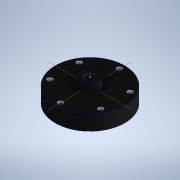
# Autodesk Inventor part: valve housing
Saved by Autodesk Inventor 2021.1 (Build 251245000, 245)
## iProperties
Created: 2020-08-29
Part Number: valve housing
Material: Aluminum 6061
Document SubType Name: Sheet Metal
Designer: Vamshi
Mass: 6082.64 g
Surface Area: 1279.34 cm^2
Volume: 2252.83 cm^3
Density: 2.7 g/cm^3
Sheet Metal Rule: Default
Appearance: Aluminum - Flat
Author: Vamshi
Autodesk Inventor part; units mm, degrees
ref_plane "YZ Plane" through (0, 0, 0) normal (1, 0, 0) x (0, 1, 0)
ref_plane "XZ Plane" through (0, 0, 0) normal (0, 1, 0) x (-1, 0, 0)
ref_plane "XY Plane" through (0, 0, 0) normal (0, 0, 1) x (1, 0, 0)
sketch "Sketch1" plane through (0, 0, 0) normal (0, 0, 1) x (1, 0, 0)
  circle A0 centre (0, 0) radius 116.84
  circle A1 centre (0, 0) radius 30.48
  dimension "d0" = 233.68
  dimension "d1" = 60.96
  constraints: 2 centre point, 2 coincident
  measures "d0" diameter of A0
  measures "d1" diameter of A1
extrude "Extrusion1" add sketch "Sketch1" against normal blind 50.8 contours A0 | A1
sketch "Sketch2" plane through (0, 0, 0) normal (0, 0, 1) x (1, 0, 0)
  circle A0 centre (0, 0) radius 30.48
  dimension "d4" = 60.96
  constraints: 1 centre point, 1 coincident
  measures "d4" diameter of A0
extrude "Extrusion2" add sketch "Sketch2" along normal blind 25.4
sketch "Sketch3" plane through (0, 0, 25.4) normal (0, 0, 1) x (1, 0, 0)
  point P0 (0, 0)
sketch "Sketch4" plane through (0, 0, 25.4) normal (0, 0, 1) x (1, 0, 0)
  circle A0 centre (0, 0) radius 6.35
  circle A1 centre (0, 0) radius 17.78
  dimension "d7" = 12.7
  dimension "d8" = 35.56
  constraints: 2 centre point, 2 coincident
  measures "d7" diameter of A0
  measures "d8" diameter of A1
extrude "Extrusion3" cut sketch "Sketch4" against normal blind 6.35 contours A0 | A1
extrude "Extrusion6" cut sketch "Sketch4" against normal through all contours A0
sketch "Sketch5" plane through (0, 0, -50.8) normal (0, 0, -1) x (-1, 0, 0)
  circle A0 centre (0, 0) radius 6.35 projected
  circle A1 centre (0, 0) radius 83.82
  dimension "d17" = 167.64
  constraints: 1 centre point, 1 coincident
  measures "d17" diameter of A1
extrude "Extrusion7" cut sketch "Sketch5" against normal blind 35.56
sketch "Sketch7" plane through (0, 0, 0) normal (1, 0, 0) x (0, 1, 0)
  circle A0 centre (0, -30.48) radius 10.16
  line L0 (-116.84, -50.8) -> (116.84, -50.8) projected
  point P0 (0, 0)
  dimension "d20" = 20.32
  dimension "d21" = 20.32
  constraints: 1 centre point
  measures "d20" diameter of A0
  measures "d21" distance from line of L0 A0.centre
extrude "Extrusion8" cut sketch "Sketch7" against normal through all
thread "Thread1" size "M8x1.25" class "6H" standard "ANSI Metric M Profile" full length
sketch "Sketch8" plane through (0, 0, 0) normal (0, 0, 1) x (1, 0, 0)
  point P0 (0, 0)
sketch "Sketch9" plane through (0, 0, 0) normal (0, 0, 1) x (1, 0, 0)
  circle A0 centre (0, 0) radius 6.35 construction
  circle A1 centre (0, 0) radius 99.06 construction
  line L0 (0, 0) -> (-123.6027, 71.3621) construction
  line L1 (0, 0) -> (-132.0824, -76.2578) construction
  line L2 (-189.6994, 0) -> (167.9299, 0) construction
  circle A2 centre (-85.7885, 49.53) radius 8.89
  circle A3 centre (-85.7885, -49.53) radius 8.89
  circle A4 centre (0, -99.06) radius 8.89
  circle A5 centre (85.7885, -49.53) radius 8.89
  circle A6 centre (85.7885, 49.53) radius 8.89
  circle A7 centre (0, 99.06) radius 8.89
  dimension "d26" = 198.12
  dimension "d27" = 60
  dimension "d28" = 17.78
  dimension "d31" = 360
  constraints: 6 centre point, 4 end point, 1 coincident, 1 point on line, 17 other
  measures "d27" angle of L1 L0
  measures "d28" diameter of A2
extrude "Extrusion9" cut sketch "Sketch9" against normal through all
thread "Thread2" size "M8x1.25" class "6H" standard "ANSI Metric M Profile" full length
equation "\"BendRadius\" = Thickness"
equation "\"BendReliefWidth\" = Thickness"
equation "\"BendReliefDepth\" = 0.5 * Thickness"
equation "\"CornerReliefSize\" = 4 * Thickness"
equation "\"MinimumRemnant\" = 2 * Thickness"
equation "\"TransitionRadius\" = BendRadius"
equation "\"JacobiRadiusSize\" = BendRadius"
equation "\"GapSize\" = Thickness"
equation "\"Thickness\" = 3.048"
body "Solid1"
